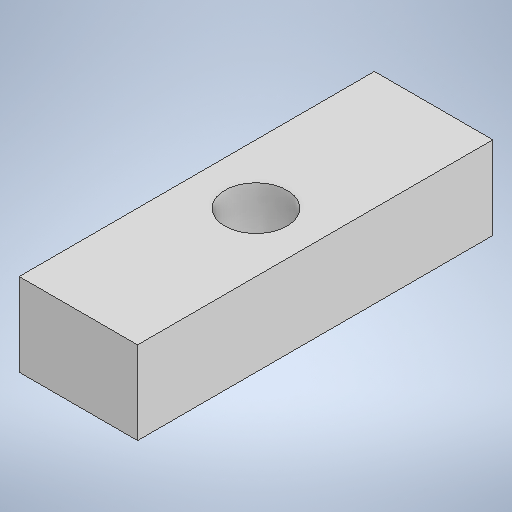
# Autodesk Inventor part: Kopf_Bruecke
Saved by Autodesk Inventor 2025 (Build 290162000, 162)
## iProperties
Created: 2026-07-13
Part Number: Kopf_Bruecke
Material: Generisch
Document SubType Name: Modeling
Designer: wavid
Mass: 14.6321 g
Surface Area: 54.1872 cm^2
Volume: 14.6321 cm^3
Density: 1 g/cm^3
Appearance: Vorgabe
Author: wavid
Autodesk Inventor part; units mm, degrees
ref_plane "YZ Plane" through (0, 0, 0) normal (1, 0, 0) x (0, 1, 0)
ref_plane "XZ Plane" through (0, 0, 0) normal (0, 1, 0) x (-1, 0, 0)
sketch "Skizze1" plane through (0, 0, 0) normal (0, 0, 1) x (1, 0, 0)
  line L0 (-10, -30) -> (10, -30)
  line L1 (10, -30) -> (10, 30)
  line L2 (10, 30) -> (-10, 30)
  line L3 (-10, 30) -> (-10, -30)
  constraints: 8 end point, 2 parallel, 1 horizontal, 1 perpendicular
extrude "Extrusion1" add sketch "Skizze1" along normal blind 14
sketch "Skizze2" plane through (0, 0, 0) normal (0, 0, 1) x (1, 0, 0)
  circle A0 centre (0, -22) radius 3.9
  constraints: 1 centre point
extrude "Extrusion2" cut sketch "Skizze2" along normal blind 10
sketch "Skizze3" plane through (0, 0, 0) normal (0, 0, 1) x (1, 0, 0)
  circle A0 centre (0, 22) radius 3.9
  constraints: 1 centre point
extrude "Extrusion3" cut sketch "Skizze3" along normal blind 10
ref_plane "Arbeitsebene1" through (0, 0, 14) normal (0, 0, 1) x (1, 0, 0)
sketch "Skizze4" plane through (0, 0, 14) normal (0, 0, 1) x (1, 0, 0)
  circle A0 centre (0, 0) radius 5.25
  constraints: 1 centre point
extrude "Extrusion4" cut sketch "Skizze4" against normal blind 14.2
